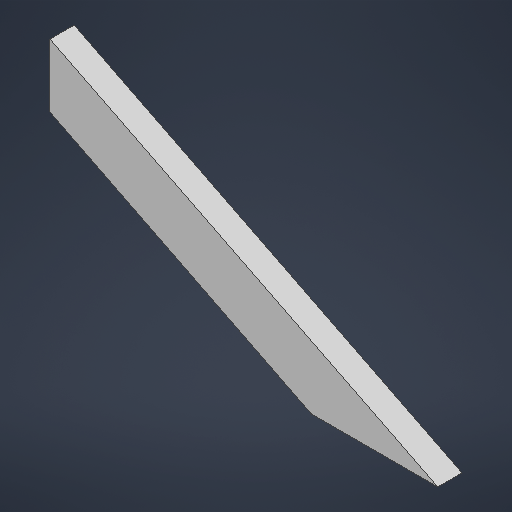
# Autodesk Inventor part: S_2x4x26.833
Saved by Autodesk Inventor 2026 (Build 300175000, 175)
## iProperties
Created: 2025-09-03
Part Number: S_2x4x26.833
Material: Generic
Document SubType Name: Modeling
Designer: trott
Density: 1 g/cm^3
Appearance: Default
Author: trott
Autodesk Inventor part; units mm, degrees
ref_plane "YZ Plane" through (0, 0, 0) normal (1, 0, 0) x (0, 1, 0)
ref_plane "XZ Plane" through (0, 0, 0) normal (0, 1, 0) x (-1, 0, 0)
ref_plane "XY Plane" through (0, 0, 0) normal (0, 0, 1) x (1, 0, 0)
sketch "Sketch1" plane through (0, 0, 0) normal (0, 0, 1) x (1, 0, 0)
  line L0 (0, 0) -> (0, 304.8)
  line L1 (0, 0) -> (609.6, 0)
  line L2 (0, 304.8) -> (609.6, 0)
  line L3 (0, 304.8) -> (-39.7573, 225.2854)
  line L4 (609.6, 0) -> (569.8427, -79.5146)
  line L5 (-39.7573, 225.2854) -> (569.8427, -79.5146)
  point P0 (0, 205.4068)
  point P1 (410.8136, 0)
  dimension "d2" = 304.8
  dimension "d3" = 609.6
  dimension "d4" = 88.9
  dimension "d5" = 90
  dimension "d6" = 88.9
  dimension "d7" = 90
  constraints: 12 end point, 1 horizontal, 1 vertical
  measures "d2" distance of L0.start L0.end
  measures "d3" distance of L0.start L1.end
  measures "d4" distance of L0.end L3.end
  measures "d5" angle of L2 L3
  measures "d6" distance of L1.end L4.end
  measures "d7" angle of L4 L2
extrude "Extrusion1" add sketch "Sketch1" along normal blind 38.1 contours L0 L2 L1 L5
body "Solid1"
